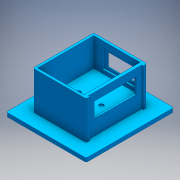
# Autodesk Inventor part: sampleChamber
Saved by Autodesk Inventor 2016 (Build 200138000, 138)
## iProperties
Created: 2016-11-09
Part Number: sampleChamber
Material: Generic
Document SubType Name: Modeling
Designer: sims01
Density: 1 g/cm^3
Appearance: Default
Author: sims01
Autodesk Inventor part; units mm, degrees
ref_plane "YZ Plane" through (0, 0, 0) normal (1, 0, 0) x (0, 1, 0)
ref_plane "XZ Plane" through (0, 0, 0) normal (0, 1, 0) x (-1, 0, 0)
ref_plane "XY Plane" through (0, 0, 0) normal (0, 0, 1) x (1, 0, 0)
sketch "Sketch1" plane through (0, 0, 0) normal (0, 0, 1) x (1, 0, 0)
  line L0 (-40.5, 47.5) -> (40.5, 47.5)
  line L1 (42.5, 45.5) -> (42.5, -45.5)
  line L2 (40.5, -47.5) -> (-40.5, -47.5)
  line L3 (-42.5, -45.5) -> (-42.5, 45.5)
  arc A0 (-40.5, 47.5) -> (-42.5, 45.5) centre (-40.5, 45.5) ccw
  arc A1 (-42.5, -45.5) -> (-40.5, -47.5) centre (-40.5, -45.5) ccw
  arc A2 (40.5, -47.5) -> (42.5, -45.5) centre (40.5, -45.5) ccw
  arc A3 (42.5, 45.5) -> (40.5, 47.5) centre (40.5, 45.5) ccw
  line L4 (-50.5, 57.5) -> (50.5, 57.5)
  line L5 (52.5, 55.5) -> (52.5, -55.5)
  line L6 (50.5, -57.5) -> (-50.5, -57.5)
  line L7 (-52.5, -55.5) -> (-52.5, 55.5)
  arc A4 (-50.5, 57.5) -> (-52.5, 55.5) centre (-50.5, 55.5) ccw
  arc A5 (-52.5, -55.5) -> (-50.5, -57.5) centre (-50.5, -55.5) ccw
  arc A6 (50.5, -57.5) -> (52.5, -55.5) centre (50.5, -55.5) ccw
  arc A7 (52.5, 55.5) -> (50.5, 57.5) centre (50.5, 55.5) ccw
  point P0 (0, 0)
  point P1 (-42.5, 47.5)
  point P2 (42.5, -47.5)
  point P3 (42.5, 47.5)
  dimension "d0" = 85
  dimension "d1" = 95
  dimension "d2" = 47.5
  dimension "d3" = 42.5
  dimension "d4" = 2
  dimension "d5" = 10
  dimension "d6" = 10
  dimension "d7" = 10
  dimension "d8" = 10
  dimension "d9" = 2
  constraints: 16 end point, 16 point on circle, 16 tangent, 8 centre point, 6 equal radius, 6 point on line, 4 parallel, 2 horizontal, 2 perpendicular
  measures "d0" distance of point (-42.5, 47.5) point (42.5, 47.5)
  measures "d1" distance of point (42.5, 47.5) point (42.5, -47.5)
  measures "d2" distance from line of point (0, 0) L0
  measures "d3" distance from line of point (0, 0) L1
  measures "d4" radius of A0
  measures "d5" distance between parallel lines of L0 L4
  measures "d6" distance between parallel lines of L7 L3
  measures "d7" distance between parallel lines of L6 L2
  measures "d8" distance between parallel lines of L5 L1
  measures "d9" radius of A4
extrude "chamberBase" add sketch "Sketch1" along normal blind 5 contours L0 A3 L1 A2 L2 A1 L3 A0 | L4 A7 L5 A6 L6 A5 L7 A4
sketch "Sketch2" plane through (0, 0, 5) normal (0, 0, 1) x (1, 0, 0)
  line L0 (-33, 40) -> (33, 40)
  line L1 (35, 38) -> (35, -38)
  line L2 (33, -40) -> (-33, -40)
  line L3 (-35, -38) -> (-35, 38)
  arc A0 (-33, 40) -> (-35, 38) centre (-33, 38) ccw
  arc A1 (-35, -38) -> (-33, -40) centre (-33, -38) ccw
  arc A2 (33, -40) -> (35, -38) centre (33, -38) ccw
  arc A3 (35, 38) -> (33, 40) centre (33, 38) ccw
  point P0 (0, 0)
  point P1 (-35, 40)
  point P2 (35, -40)
  point P3 (35, 40)
  dimension "d12" = 70
  dimension "d13" = 80
  dimension "d14" = 40
  dimension "d15" = 35
  dimension "d16" = 2
  constraints: 8 end point, 8 point on circle, 8 tangent, 6 point on line, 4 centre point, 3 equal radius, 2 parallel, 1 horizontal, 1 perpendicular
  measures "d12" distance of point (-35, 40) point (35, 40)
  measures "d13" distance of point (35, 40) point (35, -40)
  measures "d14" distance from line of point (0, 0) L0
  measures "d15" distance from line of point (0, 0) L1
  measures "d16" radius of A0
extrude "chamberWallExt" add sketch "Sketch2" along normal blind 50
sketch "Sketch3" plane through (0, 0, 55) normal (0, 0, 1) x (1, 0, 0)
  line L0 (-32, 37) -> (29, 37)
  line L1 (29, 37) -> (29, -37)
  line L2 (29, -37) -> (-32, -37)
  line L3 (-32, -37) -> (-32, 37)
  line L4 (-33, 40) -> (33, 40) projected
  line L5 (35, -38) -> (35, 38) projected
  line L6 (-33, -40) -> (33, -40) projected
  line L7 (-35, -38) -> (-35, 38) projected
  point P0 (0, 0)
  dimension "d19" = 3
  dimension "d21" = 3
  dimension "d46" = 3
  dimension "d47" = 6
  constraints: 8 end point, 2 parallel, 1 horizontal, 1 perpendicular
  measures "d19" distance between parallel lines of L4 L0
  measures "d21" distance between parallel lines of L6 L2
  measures "d46" distance between parallel lines of L7 L3
  measures "d47" distance between parallel lines of L1 L5
extrude "chamberIntExt" cut sketch "Sketch3" against normal blind 37.5
sketch "Sketch4" plane through (29, -37, 55) normal (-1, 0, 0) x (0, 0, 1)
  line L0 (-5, 69.5) -> (-35, 69.5)
  line L1 (-35, 69.5) -> (-35, 4.5)
  line L2 (-35, 4.5) -> (-5, 4.5)
  line L3 (-5, 4.5) -> (-5, 69.5)
  line L4 (-50, -18.5) -> (-50, 92.5) projected
  point P0 (-55, 37)
  dimension "d25" = 65
  dimension "d26" = 30
  dimension "d27" = 32.5
  dimension "d28" = 45
  constraints: 8 end point, 2 parallel, 1 horizontal, 1 perpendicular
  measures "d25" distance of L2.end L0.start
  measures "d26" distance of L1.end L2.end
  measures "d27" distance from line of point (-55, 37) L2
  measures "d28" distance between parallel lines of L4 L3
extrude "rectCoverSlipMountExt" cut sketch "Sketch4" against normal blind 2
sketch "Sketch5" plane through (31, -37, 55) normal (-1, 0, 0) x (0, 0, 1)
  line L0 (-10, 64.5) -> (-30, 64.5)
  line L1 (-30, 64.5) -> (-30, 9.5)
  line L2 (-30, 9.5) -> (-10, 9.5)
  line L3 (-10, 9.5) -> (-10, 64.5)
  line L4 (-50, 92.5) -> (-50, -18.5) projected
  point P0 (-55, 37)
  dimension "d31" = 55
  dimension "d32" = 20
  dimension "d33" = 27.5
  dimension "d34" = 40
  constraints: 8 end point, 2 parallel, 1 horizontal, 1 perpendicular
  measures "d31" distance of L2.end L0.start
  measures "d32" distance of L1.end L2.end
  measures "d33" distance from line of point (-55, 37) L2
  measures "d34" distance between parallel lines of L4 L3
extrude "rectCoverSlipWindow" cut sketch "Sketch5" against normal up to surface (4 mm away)
sketch "Sketch7" plane through (35, -38, 5) normal (1, 0, 0) x (0, 0, -1)
  line L0 (-50, 3) -> (0, 3)
  line L1 (0, 3) -> (0, 73)
  line L2 (0, 73) -> (-50, 73)
  line L3 (-50, 73) -> (-50, 3)
  line L4 (-50, 0) -> (-50, 76) projected
  line L5 (0, 76) -> (0, 0) projected
  point P0 (5, 38)
  dimension "d42" = 70
  dimension "d43" = 35
  constraints: 8 end point, 2 collinear, 2 parallel, 1 horizontal, 1 perpendicular
  measures "d42" distance of L2.end L0.start
  measures "d43" distance from line of point (5, 38) L2
extrude "illObjExt" cut sketch "Sketch7" against normal blind 2
sketch "Sketch8" plane through (-32, 37, 55) normal (0, -1, 0) x (1, 0, 0)
  line L0 (56.5, -32.5) -> (11.5, -32.5)
  line L1 (11.5, -32.5) -> (11.5, -7.5)
  line L2 (11.5, -7.5) -> (56.5, -7.5)
  line L3 (56.5, -7.5) -> (56.5, -32.5)
  line L4 (0, -37.5) -> (61, -37.5) projected
  line L5 (-18.5, -50) -> (82.5, -50) projected
  point P0 (32, -55)
  point P1 (61, -5)
  dimension "d48" = 25
  dimension "d49" = 45
  dimension "d52" = 42.5
  dimension "d109" = 4.5
  constraints: 8 end point, 2 parallel, 1 horizontal, 1 perpendicular
  measures "d48" distance of L2.end L0.start
  measures "d49" distance of L1.end L2.end
  measures "d52" distance between parallel lines of L5 L2
  measures "d109" distance from line of L3 point (61, -5)
extrude "viewingWindCoverSlipMount" cut sketch "Sketch8" against normal blind 2
sketch "Sketch9" plane through (-32, 39, 55) normal (0, -1, 0) x (1, 0, 0)
  line L0 (16.5, -11.5) -> (51.5, -11.5)
  line L1 (51.5, -11.5) -> (51.5, -28.5)
  line L2 (51.5, -28.5) -> (16.5, -28.5)
  line L3 (16.5, -28.5) -> (16.5, -11.5)
  line L4 (82.5, -50) -> (-18.5, -50) projected
  line L5 (56.5, -7.5) -> (56.5, -32.5) projected
  point P0 (32, -55)
  dimension "d55" = 35
  dimension "d56" = 17
  dimension "d58" = 38.5
  dimension "d110" = 5
  constraints: 8 end point, 2 parallel, 1 horizontal, 1 perpendicular
  measures "d55" distance of L0.start L0.end
  measures "d56" distance of L2.end L0.start
  measures "d58" distance between parallel lines of L4 L0
  measures "d110" distance between parallel lines of L1 L5
extrude "viewingWindExt" cut sketch "Sketch9" against normal up to surface (1 mm away)
sketch "Sketch10" plane through (0, 0, 17.5) normal (0, 0, 1) x (1, 0, 0)
  circle A0 centre (0, -15) radius 2.825
  circle A1 centre (15, 0) radius 2.825
  circle A2 centre (0, 15) radius 2.825
  circle A3 centre (-15, 0) radius 2.825
  circle A4 centre (0, 0) radius 2.825
  dimension "d70" = 5.65
  dimension "d71" = 5.65
  dimension "d72" = 5.65
  dimension "d73" = 5.65
  dimension "d74" = 5.65
  dimension "d75" = 15
  dimension "d76" = 15
  dimension "d77" = 15
  dimension "d78" = 15
  constraints: 5 centre point, 2 coincident, 2 horizontal alignment, 2 vertical alignment
  measures "d70" diameter of A1
  measures "d71" diameter of A0
  measures "d72" diameter of A2
  measures "d73" diameter of A4
  measures "d74" diameter of A3
  measures "d75" distance of A4.centre A0.centre
  measures "d76" distance of A1.centre A4.centre
  measures "d77" distance of A2.centre A4.centre
  measures "d78" distance of A3.centre A4.centre
extrude "sampleHolderMagnets" cut sketch "Sketch10" against normal blind 2
sketch "Sketch13" plane through (0, 0, 0) normal (0, 0, -1) x (-1, 0, 0)
  circle A0 centre (0, 55) radius 1.325
  circle A1 centre (-50, 0) radius 1.325
  circle A2 centre (0, -55) radius 1.325
  circle A3 centre (0, 0) radius 1.325
  circle A4 centre (50, 0) radius 1.325
  dimension "d98" = 2.65
  dimension "d99" = 2.65
  dimension "d100" = 2.65
  dimension "d101" = 2.65
  dimension "d102" = 2.65
  dimension "d103" = 55
  dimension "d104" = 55
  dimension "d105" = 50
  dimension "d106" = 50
  constraints: 5 centre point, 2 coincident, 2 horizontal alignment, 2 vertical alignment
  measures "d98" diameter of A0
  measures "d99" diameter of A2
  measures "d100" diameter of A1
  measures "d101" diameter of A3
  measures "d102" diameter of A4
  measures "d103" distance of A0.centre point (0, 0)
  measures "d104" distance of A2.centre point (0, 0)
  measures "d105" distance of A4.centre point (0, 0)
  measures "d106" distance of A1.centre point (0, 0)
extrude "xyStageMount" cut sketch "Sketch13" against normal blind 2
equation "\"d2\" = 0.5 * d1"
equation "\"d3\" = 0.5 * d0"
equation "\"d6\" = d5"
equation "\"d7\" = d5"
equation "\"d8\" = d5"
equation "\"d14\" = 0.5 * d13"
equation "\"d15\" = 0.5 * d12"
equation "\"d21\" = d19"
equation "\"d46\" = d19"
equation "\"d27\" = 0.5 * d25"
equation "\"d33\" = 0.5 * d31"
equation "\"d43\" = 0.5 * d42"
equation "\"d71\" = d70"
equation "\"d72\" = d70"
equation "\"d73\" = d70"
equation "\"d74\" = d70"
equation "\"d76\" = d75"
equation "\"d77\" = d75"
equation "\"d78\" = d75"
equation "\"d99\" = d98"
equation "\"d100\" = d98"
equation "\"d101\" = d98"
equation "\"d102\" = d98"
equation "\"d104\" = d103"
equation "\"d106\" = d105"
body "Solid1"
